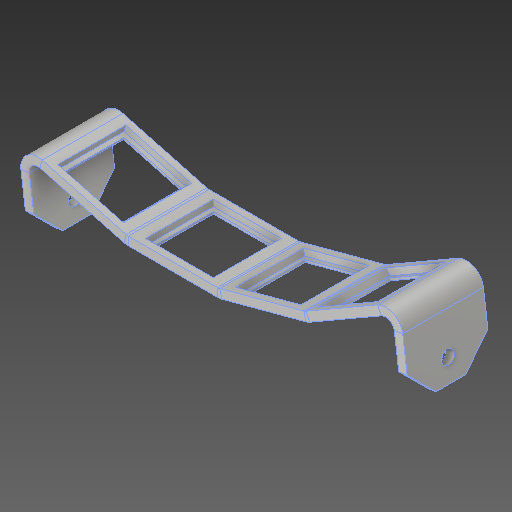
# Autodesk Inventor part: keyplate4
Saved by Autodesk Inventor 2018 (Build 220112000, 112)
## iProperties
Created: 2018-05-25
Part Number: keyplate4
Material: アルミニウム 6061
Document SubType Name: Sheet Metal
Designer: NaMACHAN
Density: 2.7 g/cm^3
Sheet Metal Rule: Al2mm
Appearance: アルミニウム - フラット
Mass: 7.00903 g
Surface Area: 40.3186 cm^2
Volume: 2.59594 cm^3
Flat Pattern Width: 1.9 cm
Flat Pattern Length: 12.3019 cm
Flat Pattern Area: 23.3736 cm^2
Sheet Metal Width: 19.000 mm
Sheet Metal Length: 123.019 mm
Sheet Metal Area: 2337.361 mm^2
Author: NaMACHAN
Autodesk Inventor part; units mm, degrees
ref_plane "YZ Plane" through (0, 0, 0) normal (1, 0, 0) x (0, 1, 0)
ref_plane "XZ Plane" through (0, 0, 0) normal (0, 1, 0) x (-1, 0, 0)
ref_plane "XY Plane" through (0, 0, 0) normal (0, 0, 1) x (1, 0, 0)
sketch "スケッチ1" plane through (0, 0, 0) normal (0, 1, 0) x (-1, 0, 0)
  line L0 (-10.5, -9.5) -> (10.5, -9.5)
  line L1 (10.5, -9.5) -> (10.5, 9.5)
  line L2 (10.5, 9.5) -> (-10.5, 9.5)
  line L3 (-10.5, 9.5) -> (-10.5, -9.5)
  line L4 (-10.5, -9.5) -> (10.5, 9.5) construction
  line L5 (10.5, -9.5) -> (-10.5, 9.5) construction
  line L6 (-7, -7) -> (7, -7)
  line L7 (7, -7) -> (7, 7)
  line L8 (7, 7) -> (-7, 7)
  line L9 (-7, 7) -> (-7, -7)
  line L10 (-7, -7) -> (7, 7) construction
  line L11 (7, -7) -> (-7, 7) construction
  point P0 (0, 0)
  dimension "d0" = 21
  dimension "d1" = 19
  dimension "d2" = 14
  dimension "d3" = 14
  measures "d0" distance of L2.end L1.end
  measures "d1" distance of L1.end L0.end
  measures "d2" distance of L8.end L7.end
  measures "d3" distance of L7.end L6.end
extrude "プレート1" add sketch "スケッチ1" along normal blind 2
sketch "スケッチ2" plane through (-11.0176, 2.0681, 9.5) normal (-0.258819, -0.9659258, 0) x (0.9659258, -0.258819, 0)
  line L0 (0, -19) -> (0, 0)
  line L1 (0, 0) -> (-20.4734, 0)
  line L2 (-20.4734, 0) -> (-20.4734, -19)
  line L3 (-20.4734, -19) -> (0, -19)
  constraints: 6 end point, 1 horizontal, 1 perpendicular, 1 vertical
edge flange "フランジ1" height 21 angle 15 thickness 2 bend radius 2 thickness toward (-0.258819, -0.9659258, 0) relief straight relief width 2 relief depth 1 edges at (-10.5, 2, 0) wall of the first edge with corners at (-11.0176, 2.0681, -9.5) (-11.0176, 2.0681, 9.5) (-30.7934, 7.3671, 9.5) (-30.7934, 7.3671, -9.5)
bend "曲げ1"
corner "コーナー1"
sketch "スケッチ3" plane through (11.0176, 2.0681, -9.5) normal (0.258819, -0.9659258, 0) x (0.9659258, 0.258819, 0)
  line L0 (0, 19) -> (0, 0)
  line L1 (0, 0) -> (20.4734, 0)
  line L2 (20.4734, 0) -> (20.4734, 19)
  line L3 (20.4734, 19) -> (0, 19)
  constraints: 6 end point, 1 horizontal, 1 perpendicular, 1 vertical
edge flange "フランジ2" height 21 angle 15 thickness 2 bend radius 2 thickness toward (0.258819, -0.9659258, 0) relief straight relief width 2 relief depth 1 edges at (10.5, 2, 0) wall of the first edge with corners at (11.0176, 2.0681, 9.5) (11.0176, 2.0681, -9.5) (30.7934, 7.3671, -9.5) (30.7934, 7.3671, 9.5)
bend "曲げ2"
corner "コーナー2"
sketch "スケッチ4" plane through (31.2758, 7.5669, -9.5) normal (0.5, -0.8660254, 0) x (0.8660254, 0.5, 0)
  line L0 (0, 19) -> (0, 0)
  line L1 (0, 0) -> (19.4734, 0)
  line L2 (19.4734, 0) -> (19.4734, 19)
  line L3 (19.4734, 19) -> (0, 19)
  constraints: 8 end point
edge flange "フランジ3" height 20 angle 15 thickness 2 bend radius 2 thickness toward (0.5, -0.8660254, 0) relief straight relief width 2 relief depth 1 edges at (30.7934, 7.3671, 0) wall of the first edge with corners at (31.2758, 7.5669, 9.5) (31.2758, 7.5669, -9.5) (48.1402, 17.3035, -9.5) (48.1402, 17.3035, 9.5)
bend "曲げ3"
corner "コーナー3"
sketch "スケッチ5" plane through (52.1231, 14.1005, -9.5) normal (0.9914449, 0.1305262, 0) x (0.1305262, -0.9914449, 0)
  line L0 (0, 19) -> (0, 0)
  line L1 (0, 0) -> (14.0136, 0)
  line L2 (14.0136, 0) -> (14.0136, 19)
  line L3 (14.0136, 19) -> (0, 19)
  constraints: 6 end point, 1 horizontal, 1 perpendicular, 1 vertical
edge flange "フランジ4" height 20 angle -112.5 thickness 2 bend radius 2 thickness toward (0.9914449, 0.1305262, 0) relief straight relief width 2 relief depth 1 edges at (48.1402, 17.3035, 0) wall of the first edge with corners at (52.1231, 14.1005, 9.5) (52.1231, 14.1005, -9.5) (53.9523, 0.2068, -9.5) (53.9523, 0.2068, 9.5)
bend "曲げ4"
corner "コーナー4"
sketch "スケッチ6" plane through (-33.8116, 3.2423, 9.5) normal (-0.9914449, -0.1305262, 0) x (-0.1305262, 0.9914449, 0)
  line L0 (0, -19) -> (0, 0)
  line L1 (0, 0) -> (-14.0136, 0)
  line L2 (-14.0136, 0) -> (-14.0136, -19)
  line L3 (-14.0136, -19) -> (0, -19)
  constraints: 6 end point, 1 horizontal, 1 perpendicular, 1 vertical
edge flange "フランジ5" height 20 angle -112.5 thickness 2 bend radius 2 thickness toward (-0.9914449, -0.1305262, 0) relief straight relief width 2 relief depth 1 edges at (-30.7934, 7.3671, 0) wall of the first edge with corners at (-33.8116, 3.2423, -9.5) (-33.8116, 3.2423, 9.5) (-31.9824, -10.6514, 9.5) (-31.9824, -10.6514, -9.5)
bend "曲げ5"
corner "コーナー5"
sketch "スケッチ7" plane through (11.0176, 2.0681, 9.5) normal (-0.258819, 0.9659258, 0) x (0.9659258, 0.258819, 0)
  line L0 (3.2367, 16.5) -> (17.2367, 16.5)
  line L1 (17.2367, 16.5) -> (17.2367, 2.5)
  line L2 (17.2367, 2.5) -> (3.2367, 2.5)
  line L3 (3.2367, 2.5) -> (3.2367, 16.5)
  line L4 (3.2367, 16.5) -> (17.2367, 2.5) construction
  line L5 (17.2367, 16.5) -> (3.2367, 2.5) construction
  line L6 (20.4734, 0) -> (0, 0) projected
  line L7 (-0.5176, 19) -> (-0.5176, 0) projected
  point P0 (-11.1775, 9.5)
  point P1 (10.2367, 9.5)
  point P2 (10.2367, 9.5)
  point P3 (10.2367, 0)
  point P4 (10.2367, 9.5)
  point P5 (-0.5176, 9.5)
  dimension "d55" = 14
  dimension "d56" = 14
  constraints: 12 end point, 6 midpoint, 2 parallel, 1 horizontal, 1 horizontal alignment, 1 perpendicular, 1 vertical alignment
  measures "d55" distance of L1.end L2.end
  measures "d56" distance of L0.end L1.end
extrude "押し出し1" cut sketch "スケッチ7" against normal blind 10
sketch "スケッチ8" plane through (31.2758, 7.5669, 9.5) normal (-0.5, 0.8660254, 0) x (0.8660254, 0.5, 0)
  line L0 (2.7367, 16.5) -> (16.7367, 16.5)
  line L1 (16.7367, 16.5) -> (16.7367, 2.5)
  line L2 (16.7367, 2.5) -> (2.7367, 2.5)
  line L3 (2.7367, 2.5) -> (2.7367, 16.5)
  line L4 (2.7367, 16.5) -> (16.7367, 2.5) construction
  line L5 (16.7367, 16.5) -> (2.7367, 2.5) construction
  line L6 (-0.5176, 0) -> (-0.5176, 19) projected
  line L7 (19.4734, 0) -> (0, 0) projected
  point P0 (-30.869, 9.5)
  point P1 (9.7367, 9.5)
  point P2 (9.7367, 9.5)
  point P3 (-0.5176, 9.5)
  point P4 (9.7367, 9.5)
  point P5 (9.7367, 0)
  dimension "d59" = 14
  dimension "d60" = 14
  constraints: 12 end point, 6 midpoint, 2 parallel, 1 horizontal, 1 horizontal alignment, 1 perpendicular, 1 vertical alignment
  measures "d59" distance of L1.end L2.end
  measures "d60" distance of L0.end L1.end
extrude "押し出し2" cut sketch "スケッチ8" against normal blind 10
sketch "スケッチ9" plane through (-11.0176, 2.0681, 9.5) normal (0.258819, 0.9659258, 0) x (0.9659258, -0.258819, 0)
  line L0 (-17.2367, 16.5) -> (-3.2367, 16.5)
  line L1 (-3.2367, 16.5) -> (-3.2367, 2.5)
  line L2 (-3.2367, 2.5) -> (-17.2367, 2.5)
  line L3 (-17.2367, 2.5) -> (-17.2367, 16.5)
  line L4 (-17.2367, 16.5) -> (-3.2367, 2.5) construction
  line L5 (-3.2367, 16.5) -> (-17.2367, 2.5) construction
  line L6 (-20.4734, 19) -> (-20.4734, 0) projected
  line L7 (-20.4734, 0) -> (0, 0) projected
  point P0 (11.1775, 9.5)
  point P1 (-10.2367, 9.5)
  point P2 (-10.2367, 9.5)
  point P3 (-20.4734, 9.5)
  point P4 (-10.2367, 9.5)
  point P5 (-10.2367, 0)
  dimension "d63" = 14
  dimension "d64" = 14
  constraints: 12 end point, 6 midpoint, 2 parallel, 1 horizontal, 1 horizontal alignment, 1 perpendicular, 1 vertical alignment
  measures "d63" distance of L1.end L2.end
  measures "d64" distance of L0.end L1.end
extrude "押し出し3" cut sketch "スケッチ9" against normal blind 10
sketch "スケッチ26" plane through (-11.0176, 2.0681, 9.5) normal (0.258819, 0.9659258, 0) x (0.9659258, -0.258819, 0)
  line L0 (-2.2367, 17.5) -> (-18.2367, 17.5)
  line L1 (-18.2367, 17.5) -> (-18.2367, 1.5)
  line L2 (-18.2367, 1.5) -> (-2.2367, 1.5)
  line L3 (-2.2367, 1.5) -> (-2.2367, 17.5)
  line L4 (-2.2367, 17.5) -> (-18.2367, 1.5) construction
  line L5 (-18.2367, 17.5) -> (-2.2367, 1.5) construction
  line L6 (-22.3211, 19) -> (-22.3211, 0) projected
  line L7 (-20.4734, 19) -> (0, 19) projected
  point P0 (11.1775, 9.5)
  point P1 (-10.2367, 9.5)
  point P2 (-10.2367, 9.5)
  point P3 (-22.3211, 9.5)
  point P4 (-10.2367, 9.5)
  point P5 (-10.2367, 17.5)
  point P6 (-10.2367, 19)
  dimension "d191" = 16
  dimension "d192" = 16
  constraints: 12 end point, 7 midpoint, 2 parallel, 2 vertical alignment, 1 horizontal, 1 horizontal alignment, 1 perpendicular
  measures "d191" distance of L2.end L1.end
  measures "d192" distance of L1.end L0.end
extrude "押し出し10" cut sketch "スケッチ26" against normal blind 1.5
sketch "スケッチ27" plane through (0, 2, 0) normal (0, 1, 0) x (1, 0, 0)
  line L0 (8, 8) -> (-8, 8)
  line L1 (-8, 8) -> (-8, -8)
  line L2 (-8, -8) -> (8, -8)
  line L3 (8, -8) -> (8, 8)
  line L4 (8, 8) -> (-8, -8) construction
  line L5 (-8, 8) -> (8, -8) construction
  point P0 (0, 0)
  dimension "d195" = 16
  dimension "d196" = 16
  constraints: 12 end point, 2 midpoint, 2 parallel, 1 horizontal, 1 perpendicular
  measures "d195" distance of L2.end L1.end
  measures "d196" distance of L1.end L0.end
extrude "押し出し11" cut sketch "スケッチ27" against normal blind 1.5
sketch "スケッチ28" plane through (11.0176, 2.0681, 9.5) normal (-0.258819, 0.9659258, 0) x (0.9659258, 0.258819, 0)
  line L0 (18.2367, 17.5) -> (2.2367, 17.5)
  line L1 (2.2367, 17.5) -> (2.2367, 1.5)
  line L2 (2.2367, 1.5) -> (18.2367, 1.5)
  line L3 (18.2367, 1.5) -> (18.2367, 17.5)
  line L4 (18.2367, 17.5) -> (2.2367, 1.5) construction
  line L5 (2.2367, 17.5) -> (18.2367, 1.5) construction
  line L6 (-0.5176, 19) -> (-0.5176, 0) projected
  line L7 (20.4734, 19) -> (0, 19) projected
  point P0 (-11.1775, 9.5)
  point P1 (10.2367, 9.5)
  point P2 (10.2367, 9.5)
  point P3 (-0.5176, 9.5)
  point P4 (10.2367, 9.5)
  point P5 (10.2367, 19)
  dimension "d199" = 16
  dimension "d200" = 16
  constraints: 12 end point, 6 midpoint, 2 parallel, 1 horizontal, 1 horizontal alignment, 1 perpendicular, 1 vertical alignment
  measures "d199" distance of L2.end L1.end
  measures "d200" distance of L1.end L0.end
extrude "押し出し12" cut sketch "スケッチ28" against normal blind 1.5
sketch "スケッチ29" plane through (31.2758, 7.5669, 9.5) normal (-0.5, 0.8660254, 0) x (0.8660254, 0.5, 0)
  line L0 (17.7367, 17.5) -> (1.7367, 17.5)
  line L1 (1.7367, 17.5) -> (1.7367, 1.5)
  line L2 (1.7367, 1.5) -> (17.7367, 1.5)
  line L3 (17.7367, 1.5) -> (17.7367, 17.5)
  line L4 (17.7367, 17.5) -> (1.7367, 1.5) construction
  line L5 (1.7367, 17.5) -> (17.7367, 1.5) construction
  line L6 (0, 19) -> (0, 0) projected
  line L7 (19.4734, 19) -> (0, 19) projected
  point P0 (-30.869, 9.5)
  point P1 (9.7367, 9.5)
  point P2 (9.7367, 9.5)
  point P3 (0, 9.5)
  point P4 (9.7367, 9.5)
  point P5 (9.7367, 17.5)
  point P6 (9.7367, 19)
  dimension "d203" = 16
  dimension "d204" = 16
  constraints: 12 end point, 7 midpoint, 2 parallel, 2 vertical alignment, 1 horizontal, 1 horizontal alignment, 1 perpendicular
  measures "d203" distance of L2.end L1.end
  measures "d204" distance of L1.end L0.end
extrude "押し出し13" cut sketch "スケッチ29" against normal blind 1.5
sketch "スケッチ30" plane through (55.9351, 0.4679, 9.5) normal (0.9914449, 0.1305262, 0) x (0, 0, -1)
  line L0 (0, 0) -> (19, 0) projected
  point P0 (9.5, 6.8371)
  point P1 (9.5, 5)
  point P2 (9.5, 0)
  dimension "d207" = 5
  constraints: 1 midpoint, 1 vertical alignment
  measures "d207" distance from line of L0 point (9.5, 5)
hole "穴4" at (55.2825, 5.4251, 0) direction (-0.9914449, -0.1305262, 0) diameter 3 depth 2 tip angle 118
sketch "スケッチ31" plane through (-33.9653, -10.9124, -9.5) normal (-0.9914449, -0.1305262, 0) x (0, 0, 1)
  circle A0 centre (9.5, 4.5486) radius 1.5 projected
  point P0 (9.5, 6.3857)
hole "穴5" at (-34.559, -6.4028, 0) direction (0.9914449, 0.1305262, 0) diameter 3 depth 2 tip angle 118
chamfer "コーナー面取り1" distance 6 angle 45 2 edges at (54.9437, 0.3373, -9.5) (54.9437, 0.3373, 9.5)
chamfer "コーナー面取り2" distance 6 angle 45 2 edges at (-32.9739, -10.7819, -9.5) (-32.9739, -10.7819, 9.5)
equation "\"d213\" = Thickness"
equation "\"d220\" = Thickness"
equation "\"d4\" = Thickness"
equation "\"d5\" = BendReliefWidth"
equation "\"d6\" = BendReliefDepth"
equation "\"d7\" = MinimumRemnant"
equation "\"d8\" = TransitionRadius"
equation "\"d11\" = BendRadius"
equation "\"d12\" = CornerReliefSize"
equation "\"d13\" = GapSize"
equation "\"d14\" = JacobiRadiusSize"
equation "\"d15\" = BendReliefWidth"
equation "\"d16\" = BendReliefDepth"
equation "\"d17\" = MinimumRemnant"
equation "\"d18\" = TransitionRadius"
equation "\"d21\" = BendRadius"
equation "\"d22\" = CornerReliefSize"
equation "\"d23\" = GapSize"
equation "\"d24\" = JacobiRadiusSize"
equation "\"d25\" = BendReliefWidth"
equation "\"d26\" = BendReliefDepth"
equation "\"d27\" = MinimumRemnant"
equation "\"d28\" = TransitionRadius"
equation "\"d31\" = BendRadius"
equation "\"d32\" = CornerReliefSize"
equation "\"d33\" = GapSize"
equation "\"d34\" = JacobiRadiusSize"
equation "\"d35\" = BendReliefWidth"
equation "\"d36\" = BendReliefDepth"
equation "\"d37\" = MinimumRemnant"
equation "\"d38\" = TransitionRadius"
equation "\"d41\" = BendRadius"
equation "\"d42\" = CornerReliefSize"
equation "\"d43\" = GapSize"
equation "\"d44\" = JacobiRadiusSize"
equation "\"d45\" = BendReliefWidth"
equation "\"d46\" = BendReliefDepth"
equation "\"d47\" = MinimumRemnant"
equation "\"d48\" = TransitionRadius"
equation "\"d51\" = BendRadius"
equation "\"d52\" = CornerReliefSize"
equation "\"d53\" = GapSize"
equation "\"d54\" = JacobiRadiusSize"
equation "\"BendRadius\" = Thickness"
equation "\"BendReliefWidth\" = Thickness"
equation "\"BendReliefDepth\" = 0.5 * Thickness"
equation "\"CornerReliefSize\" = 4 * Thickness"
equation "\"MinimumRemnant\" = 2 * Thickness"
equation "\"TransitionRadius\" = BendRadius"
equation "\"JacobiRadiusSize\" = BendRadius"
equation "\"GapSize\" = Thickness"
equation "\"Thickness\" = 2"
